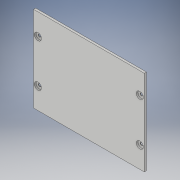
# Autodesk Inventor part: Ra-Manager_Painel_Placas-Cego
Saved by Autodesk Inventor 2019.4 (Build 234330000, 330)
## iProperties
Created: 2020-03-23
Part Number: Ra-Manager_Painel_Placas-Cego
Material: Genérico
Document SubType Name: Modeling
Designer: caiom
Density: 1 g/cm^3
Appearance: Padrão
Author: caiom
Autodesk Inventor part; units mm, degrees
ref_plane "YZ Plane" through (0, 0, 0) normal (1, 0, 0) x (0, 1, 0)
ref_plane "XZ Plane" through (0, 0, 0) normal (0, 1, 0) x (-1, 0, 0)
ref_plane "XY Plane" through (0, 0, 0) normal (0, 0, 1) x (1, 0, 0)
sketch "Esboço1" plane through (0, 0, 0) normal (0, 0, 1) x (1, 0, 0)
  line L0 (50.5, 39) -> (-50.5, 39)
  line L1 (-50.5, 39) -> (-50.5, -39)
  line L2 (-50.5, -39) -> (50.5, -39)
  line L3 (50.5, 39) -> (50.5, -39)
  point P0 (0, 0)
  dimension "d2" = 101
  dimension "d3" = 78
  dimension "d4" = 50.5
  dimension "d5" = 39
  constraints: 8 end point, 2 perpendicular, 1 parallel, 1 vertical
  measures "d2" distance of L0.start L0.end
  measures "d3" distance of L0.end L1.end
  measures "d4" distance from line of point (0, 0) L3
  measures "d5" distance from line of point (0, 0) L0
extrude "Extrusão1" add sketch "Esboço1" against normal blind 2
sketch "Esboço2" plane through (0, 0, 0) normal (0, 0, 1) x (1, 0, 0)
  line L0 (-50.5, 39) -> (50.5, 39) projected
  line L1 (-42.5, 39) -> (-42.5, -39.1132) construction
  line L2 (42.5, 39) -> (42.5, -39.1132) construction
  line L3 (-50.5, 19.5) -> (50.5, 19.5) construction
  line L4 (-50.5, -39) -> (-50.5, 39) projected
  line L5 (-50.5, -19.6132) -> (50.5, -19.6132) construction
  line L6 (-46.5, 39) -> (-46.5, -39) construction
  line L7 (50.5, -39) -> (-50.5, -39) projected
  line L8 (46.5, 39) -> (46.5, -39) construction
  point P0 (0, 0)
  point P1 (-46.5, 19.5)
  point P2 (-46.5, -19.6132)
  point P3 (46.5, -19.6132)
  point P4 (46.5, 19.5)
  constraints: 15 point on line, 12 end point, 3 vertical, 2 horizontal, 1 perpendicular
hole "Furo1" at (-46.5, 19.5, 0) at (-46.5, -19.6132, 0) at (46.5, -19.6132, 0) at (46.5, 19.5, 0) direction (0, 0, -1) diameter 2.459 end through all counterbore diameter 6.5 counterbore depth 1.5 thread size "M3x0.5" class "6H" standard "ANSI Metric M Profile"
